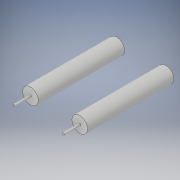
# Autodesk Inventor part: endOfArm
Saved by Autodesk Inventor 2018.2 (Build 222227000, 227)
## iProperties
Created: 2018-02-13
Part Number: endOfArm
Material: Generic
Document SubType Name: Modeling
Designer: steele
Density: 1 g/cm^3
Appearance: Default
Author: steele
Autodesk Inventor part; units mm, degrees
ref_plane "YZ Plane" through (0, 0, 0) normal (1, 0, 0) x (0, 1, 0)
ref_plane "XZ Plane" through (0, 0, 0) normal (0, 1, 0) x (-1, 0, 0)
ref_plane "XY Plane" through (0, 0, 0) normal (0, 0, 1) x (1, 0, 0)
sketch "Sketch1" plane through (0, 0, 0) normal (0, 0, 1) x (1, 0, 0)
  circle A0 centre (-76.2, 0) radius 19.05
  circle A1 centre (-76.2, 0) radius 24.13
  line L0 (0, 0) -> (0, 45.2549) construction
  circle A2 centre (76.2, 0) radius 19.05
  circle A3 centre (76.2, 0) radius 24.13
  dimension "d0" = 38.1
  dimension "d1" = 76.2
  dimension "d2" = 48.26
  constraints: 4 centre point, 2 coincident, 2 end point, 2 symmetric about line, 1 vertical, 2 other
  measures "d0" diameter of A0
  measures "d1" distance of L0.start A0.centre
  measures "d2" diameter of A1
extrude "Extrusion1" add sketch "Sketch1" against normal blind 254
sketch "Sketch2" plane through (-76.2, 0, 0) normal (0, 0, 1) x (1, 0, 0)
  circle A0 centre (0, 0) radius 24.13
  circle A1 centre (152.4, 0) radius 19.05 projected
  circle A2 centre (152.4, 0) radius 24.13
  point P0 (76.2, 0)
  constraints: 2 centre point, 1 coincident
extrude "Extrusion3" add sketch "Sketch2" along normal blind 12.7 contours A0 | A1 | A2
sketch "Sketch3" plane through (-76.2, 0, 12.7) normal (0, 0, 1) x (1, 0, 0)
  circle A0 centre (0, 0) radius 3.175
  circle A1 centre (152.4, 0) radius 19.05 projected
  circle A2 centre (152.4, 0) radius 3.175
  point P0 (76.2, 0)
  dimension "d9" = 6.35
  dimension "d10" = 6.35
  constraints: 2 centre point, 1 coincident
  measures "d9" diameter of A0
  measures "d10" diameter of A2
extrude "Extrusion4" add sketch "Sketch3" along normal blind 50.8 contours A0 | A2
body "Solid1"
